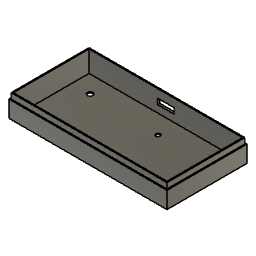
fond_boitier (Autodesk Fusion 360 design; units mm, degrees)
Autodesk Fusion 360 part; units mm, degrees
sketch "Esquisse1" plane through (0, 0, 0) normal (0, 0, 1) x (1, 0, 0)
  line L0 (70, 50) -> (-70, 50)
  line L1 (-70, 50) -> (-70, -20)
  line L2 (-70, -20) -> (70, -20)
  line L3 (70, -20) -> (70, 50)
  dimension "d1" = 140
  dimension "d2" = 70
  constraint horizontal L0
  constraint vertical L1
  constraint horizontal L2
  constraint vertical L3
  measures "d1" distance of L0.start L0.end
  measures "d2" distance of L0.start L2.end
extrude "Extrusion1" add sketch "Esquisse1" along normal blind 20
sketch "Esquisse2" plane through (0, 0, 20) normal (0, 0, 1) x (-1, 0, 0)
  line L0 (-70, 20) -> (-70, -50)
  line L1 (-70, -50) -> (70, -50)
  line L2 (70, -50) -> (70, 20)
  line L3 (70, 20) -> (-70, 20)
  line L4 (69, -49) -> (-69, -49)
  line L5 (-69, -49) -> (-69, 19)
  line L6 (-69, 19) -> (69, 19)
  line L7 (69, 19) -> (69, -49)
  constraint horizontal L4
  constraint vertical L5
  constraint horizontal L6
  constraint vertical L7
extrude "Extrusion2" cut sketch "Esquisse2" against normal blind 19 contours L4 L5 L6 L7
sketch "Esquisse3" plane through (0, 0, 1) normal (0, 0, 1) x (-1, 0, 0)
  line L0 (69, 19) -> (-69, 19)
  line L1 (-69, 19) -> (-69, -49)
  line L2 (-69, -49) -> (69, -49)
  line L3 (69, -49) -> (69, 19)
  line L4 (60, -30) -> (45, -30)
  line L5 (45, -30) -> (45, 0)
  line L6 (45, 0) -> (60, 0)
  line L7 (60, 0) -> (60, -30)
  line L8 (-60, -30) -> (-45, -30)
  line L9 (-45, -30) -> (-45, 0)
  line L10 (-45, 0) -> (-60, 0)
  line L11 (-60, 0) -> (-60, -30)
  circle A0 centre (-52.5, 3.5) radius 2.5
  circle A1 centre (-52.5, -33.4839) radius 2.5
  circle A2 centre (52.5, 3.5) radius 2.5
  circle A3 centre (52.5, -33.5) radius 2.5
  dimension "d7" = 5
  dimension "d8" = 5
  dimension "d9" = 5
  dimension "d10" = 5
  constraint horizontal L4
  constraint vertical L5
  constraint horizontal L6
  constraint vertical L7
  constraint horizontal L8
  constraint vertical L9
  constraint horizontal L10
  constraint vertical L11
  measures "d7" diameter of A0
  measures "d8" diameter of A1
  measures "d9" diameter of A2
  measures "d10" diameter of A3
extrude "Extrusion3" cut sketch "Esquisse3" against normal blind 1 contours A0 | A1 | A2 | A3
sketch "Esquisse4" plane through (0, 0, 1) normal (0, 0, 1) x (-1, 0, 0)
  circle A0 centre (52.5, 3.5) radius 2.5
  circle A1 centre (-52.5, 3.5) radius 2.5
  circle A2 centre (52.5, -33.5) radius 2.5
  circle A3 centre (-52.5, -33.4839) radius 2.5
  line L0 (69, 19) -> (-69, 19)
  line L1 (-69, 19) -> (-69, -49)
  line L2 (-69, -49) -> (69, -49)
  line L3 (69, -49) -> (69, 19)
  line L4 (12.278, -35) -> (-12.722, -35)
  line L5 (-12.722, -35) -> (-12.722, 0)
  line L6 (-12.722, 0) -> (12.278, 0)
  line L7 (12.278, 0) -> (12.278, -35)
  circle A4 centre (-10, -32) radius 2
  dimension "d13" = 25
  dimension "d14" = 35
  dimension "d16" = 4
  constraint horizontal L4
  constraint vertical L5
  constraint horizontal L6
  constraint vertical L7
  measures "d13" distance of L4.start L4.end
  measures "d14" distance of L4.start L6.end
  measures "d16" diameter of A4
extrude "Extrusion4" cut sketch "Esquisse4" against normal blind 1 contours A4
sketch "Esquisse5" plane through (0, 50, 0) normal (0, 1, 0) x (-1, 0, 0)
  line L0 (-70, 0) -> (70, 0)
  line L1 (70, 0) -> (70, 20)
  line L2 (70, 20) -> (-70, 20)
  line L3 (-70, 20) -> (-70, 0)
  line L4 (7.5, 7.5) -> (-7.5, 7.5)
  line L5 (-7.5, 7.5) -> (-7.5, 12.5)
  line L6 (-7.5, 12.5) -> (7.5, 12.5)
  line L7 (7.5, 12.5) -> (7.5, 7.5)
  constraint horizontal L4
  constraint vertical L5
  constraint horizontal L6
  constraint vertical L7
extrude "Extrusion5" cut sketch "Esquisse5" against normal blind 1 contours L4 L5 L6 L7
sketch "Esquisse6" plane through (0, 0, 0) normal (0, 0, 1) x (1, 0, 0)
  line L0 (-71, 51) -> (71, 51)
  line L1 (71, 51) -> (71, -21)
  line L2 (71, -21) -> (-71, -21)
  line L3 (-71, -21) -> (-71, 51)
  constraint horizontal L0
  constraint vertical L1
  constraint horizontal L2
  constraint vertical L3
extrude "Extrusion6" add sketch "Esquisse6" along normal blind 15 thin wall 1 inside
extrude "Extrusion7" cut 1 faces at (-2.5, 50, 9.1667) along direction (0, 1, 0) blind 1
